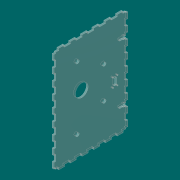
# Autodesk Inventor part: leftSide
Saved by Autodesk Inventor 2016 (Build 200138000, 138)
## iProperties
Created: 2015-10-05
Part Number: leftSide
Material: Polycarbonate, Clear
Document SubType Name: Modeling
Designer: Sawaiz
Density: 1.2 g/cm^3
Appearance: Polycarbonate - Clear
Author: Sawaiz
Autodesk Inventor part; units mm, degrees
ref_plane "YZ Plane" through (0, 0, 0) normal (1, 0, 0) x (0, 1, 0)
ref_plane "XZ Plane" through (0, 0, 0) normal (0, 1, 0) x (-1, 0, 0)
ref_plane "XY Plane" through (0, 0, 0) normal (0, 0, 1) x (1, 0, 0)
sketch "Sketch1" plane through (0, 0, 0) normal (1, 0, 0) x (0, 1, 0)
  line L0 (-60, -86.825) -> (60, -86.825)
  line L1 (60, -86.825) -> (60, 86.825)
  line L2 (60, 86.825) -> (-60, 86.825)
  line L3 (-60, 86.825) -> (-60, -86.825)
  line L4 (-60, -86.825) -> (60, 86.825) construction
  line L5 (60, -86.825) -> (-60, 86.825) construction
  point P0 (0, 0)
  dimension "d0" = 120
  dimension "d1" = 173.65
  constraints: 12 end point, 2 midpoint, 2 parallel, 1 horizontal, 1 perpendicular
  measures "d0" distance of L2.end L1.end
  measures "d1" distance of L1.end L0.end
extrude "Extrusion1" add sketch "Sketch1" along normal blind 3.175
sketch "Sketch10" plane through (0, 0, 0) normal (-1, 0, 0) x (0, 0, 1)
  line L0 (-86.825, -60) -> (-86.825, 60) projected
  line L1 (86.825, -60) -> (-86.825, -60) projected
  line L2 (86.825, 60) -> (86.825, -60) projected
  line L3 (-86.825, 60) -> (86.825, 60) projected
  line L4 (86.825, 60) -> (86.825, -60) projected
  line L5 (86.825, -55) -> (90, -55)
  line L6 (90, -55) -> (90, -45)
  line L7 (90, -45) -> (86.825, -45)
  line L8 (86.825, -45) -> (86.825, -55)
  point P0 (0, 0)
  dimension "d84" = 10
  dimension "d85" = 5
  dimension "d86" = 3.175
  constraints: 8 end point, 2 parallel, 1 horizontal, 1 perpendicular, 1 point on line
  measures "d84" distance of L5.end L6.end
  measures "d85" distance between parallel lines of L1 L5
  measures "d86" distance of L6.end L7.end
extrude "Extrusion4" add sketch "Sketch10" against normal up to surface (3.175 mm away) contours L2 L7 L6 L5
pattern_linear "Rectangular Pattern3" count 6 spacing 20 along (0, 1, 0) of "Extrusion4"
mirror "Mirror3" about plane through (0, 0, 0) normal (0, 0, 1) of "Extrusion4", "Rectangular Pattern3"
sketch "Sketch11" plane through (0, 0, 0) normal (-1, 0, 0) x (0, 0, 1)
  line L0 (-86.825, -60) -> (-86.825, -55) projected
  line L1 (86.825, -60) -> (-86.825, -60) projected
  line L2 (86.825, -55) -> (86.825, -60) projected
  line L3 (86.825, -55) -> (90, -55) projected
  line L4 (90, -55) -> (90, -45) projected
  line L5 (90, -45) -> (86.825, -45) projected
  line L6 (86.825, -35) -> (86.825, -45) projected
  line L7 (86.825, -35) -> (90, -35) projected
  line L8 (90, -35) -> (90, -25) projected
  line L9 (90, -25) -> (86.825, -25) projected
  line L10 (86.825, -15) -> (86.825, -25) projected
  line L11 (86.825, -15) -> (90, -15) projected
  line L12 (90, -15) -> (90, -5) projected
  line L13 (90, -5) -> (86.825, -5) projected
  line L14 (86.825, 5) -> (86.825, -5) projected
  line L15 (86.825, 5) -> (90, 5) projected
  line L16 (90, 5) -> (90, 15) projected
  line L17 (90, 15) -> (86.825, 15) projected
  line L18 (86.825, 25) -> (86.825, 15) projected
  line L19 (86.825, 25) -> (90, 25) projected
  line L20 (90, 25) -> (90, 35) projected
  line L21 (90, 35) -> (86.825, 35) projected
  line L22 (86.825, 45) -> (86.825, 35) projected
  line L23 (86.825, 45) -> (90, 45) projected
  line L24 (90, 45) -> (90, 55) projected
  line L25 (90, 55) -> (86.825, 55) projected
  line L26 (86.825, 60) -> (86.825, 55) projected
  line L27 (-86.825, 60) -> (86.825, 60) projected
  line L28 (-86.825, 55) -> (-86.825, 60) projected
  line L29 (-90, 55) -> (-86.825, 55) projected
  line L30 (-90, 45) -> (-90, 55) projected
  line L31 (-86.825, 45) -> (-90, 45) projected
  line L32 (-86.825, 35) -> (-86.825, 45) projected
  line L33 (-90, 35) -> (-86.825, 35) projected
  line L34 (-90, 25) -> (-90, 35) projected
  line L35 (-86.825, 25) -> (-90, 25) projected
  line L36 (-86.825, 15) -> (-86.825, 25) projected
  line L37 (-90, 15) -> (-86.825, 15) projected
  line L38 (-90, 5) -> (-90, 15) projected
  line L39 (-86.825, 5) -> (-90, 5) projected
  line L40 (-86.825, -5) -> (-86.825, 5) projected
  line L41 (-90, -5) -> (-86.825, -5) projected
  line L42 (-90, -15) -> (-90, -5) projected
  line L43 (-86.825, -15) -> (-90, -15) projected
  line L44 (-86.825, -25) -> (-86.825, -15) projected
  line L45 (-90, -25) -> (-86.825, -25) projected
  line L46 (-90, -35) -> (-90, -25) projected
  line L47 (-86.825, -35) -> (-90, -35) projected
  line L48 (-86.825, -45) -> (-86.825, -35) projected
  line L49 (-90, -45) -> (-86.825, -45) projected
  line L50 (-90, -55) -> (-90, -45) projected
  line L51 (-86.825, -55) -> (-90, -55) projected
  line L52 (86.825, -60) -> (-86.825, -60) projected
  line L53 (85, -60) -> (75, -60)
  line L54 (75, -60) -> (75, -63.175)
  line L55 (75, -63.175) -> (85, -63.175)
  line L56 (85, -63.175) -> (85, -60)
  point P0 (0, 0)
  dimension "d92" = 3.175
  dimension "d94" = 10
  dimension "d100" = 5
  constraints: 8 end point, 2 parallel, 1 horizontal, 1 perpendicular, 1 point on line
  measures "d92" distance of L55.end L53.start
  measures "d94" distance of L54.end L55.end
  measures "d100" distance between parallel lines of L4 L56
extrude "Extrusion5" add sketch "Sketch11" against normal up to surface (3.175 mm away) contours L1 L56 L55 L54
pattern_linear "Rectangular Pattern4" count 9 spacing 20 along (0, 0, -1) of "Extrusion5"
mirror "Mirror4" about plane through (0, 0, 0) normal (0, 1, 0) of "Extrusion5", "Rectangular Pattern4"
sketch "Sketch2" plane through (3.175, 0, 0) normal (1, 0, 0) x (0, 0, -1)
  line L0 (86.825, -60) -> (86.825, -55) projected
  line L1 (86.825, 60) -> (85, 60) projected
  line L2 (-86.825, 60) -> (-86.825, 55) projected
  line L3 (-86.825, -60) -> (-85, -60) projected
  line L4 (-86.825, 60) -> (-86.825, -60) projected
  line L5 (86.825, -55) -> (90, -55) projected
  line L6 (90, -55) -> (90, -45) projected
  line L7 (90, -45) -> (86.825, -45) projected
  line L8 (86.825, -45) -> (86.825, -35) projected
  line L9 (86.825, -35) -> (90, -35) projected
  line L10 (90, -35) -> (90, -25) projected
  line L11 (90, -25) -> (86.825, -25) projected
  line L12 (86.825, -25) -> (86.825, -15) projected
  line L13 (86.825, -15) -> (90, -15) projected
  line L14 (90, -15) -> (90, -5) projected
  line L15 (90, -5) -> (86.825, -5) projected
  line L16 (86.825, -5) -> (86.825, 5) projected
  line L17 (86.825, 5) -> (90, 5) projected
  line L18 (90, 5) -> (90, 15) projected
  line L19 (90, 15) -> (86.825, 15) projected
  line L20 (86.825, 15) -> (86.825, 25) projected
  line L21 (86.825, 25) -> (90, 25) projected
  line L22 (90, 25) -> (90, 35) projected
  line L23 (90, 35) -> (86.825, 35) projected
  line L24 (86.825, 35) -> (86.825, 45) projected
  line L25 (86.825, 45) -> (90, 45) projected
  line L26 (90, 45) -> (90, 55) projected
  line L27 (90, 55) -> (86.825, 55) projected
  line L28 (86.825, 55) -> (86.825, 60) projected
  line L29 (85, 60) -> (85, 63.175) projected
  line L30 (85, 63.175) -> (75, 63.175) projected
  line L31 (75, 63.175) -> (75, 60) projected
  line L32 (65, 60) -> (65, 63.175) projected
  line L33 (65, 63.175) -> (55, 63.175) projected
  line L34 (55, 63.175) -> (55, 60) projected
  line L35 (55, 60) -> (45, 60) projected
  line L36 (45, 60) -> (45, 63.175) projected
  line L37 (45, 63.175) -> (35, 63.175) projected
  line L38 (35, 63.175) -> (35, 60) projected
  line L39 (35, 60) -> (25, 60) projected
  line L40 (25, 60) -> (25, 63.175) projected
  line L41 (25, 63.175) -> (15, 63.175) projected
  line L42 (15, 63.175) -> (15, 60) projected
  line L43 (15, 60) -> (5, 60) projected
  line L44 (5, 60) -> (5, 63.175) projected
  line L45 (5, 63.175) -> (-5, 63.175) projected
  line L46 (-5, 63.175) -> (-5, 60) projected
  line L47 (-5, 60) -> (-15, 60) projected
  line L48 (-15, 60) -> (-15, 63.175) projected
  line L49 (-15, 63.175) -> (-25, 63.175) projected
  line L50 (-25, 63.175) -> (-25, 60) projected
  line L51 (-25, 60) -> (-35, 60) projected
  line L52 (-35, 60) -> (-35, 63.175) projected
  line L53 (-35, 63.175) -> (-45, 63.175) projected
  line L54 (-45, 63.175) -> (-45, 60) projected
  line L55 (-45, 60) -> (-55, 60) projected
  line L56 (-55, 60) -> (-55, 63.175) projected
  line L57 (-55, 63.175) -> (-65, 63.175) projected
  line L58 (-65, 63.175) -> (-65, 60) projected
  line L59 (-65, 60) -> (-75, 60) projected
  line L60 (-75, 60) -> (-75, 63.175) projected
  line L61 (-75, 63.175) -> (-85, 63.175) projected
  line L62 (-85, 63.175) -> (-85, 60) projected
  line L63 (-85, 60) -> (-86.825, 60) projected
  line L64 (-90, 55) -> (-86.825, 55) projected
  line L65 (-90, 45) -> (-90, 55) projected
  line L66 (-86.825, 45) -> (-90, 45) projected
  line L67 (-86.825, 45) -> (-86.825, 35) projected
  line L68 (-90, 35) -> (-86.825, 35) projected
  line L69 (-90, 25) -> (-90, 35) projected
  line L70 (-86.825, 25) -> (-90, 25) projected
  line L71 (-86.825, 25) -> (-86.825, 15) projected
  line L72 (-90, 15) -> (-86.825, 15) projected
  line L73 (-90, 5) -> (-90, 15) projected
  line L74 (-86.825, 5) -> (-90, 5) projected
  line L75 (-86.825, 5) -> (-86.825, -5) projected
  line L76 (-90, -5) -> (-86.825, -5) projected
  line L77 (-90, -15) -> (-90, -5) projected
  line L78 (-86.825, -15) -> (-90, -15) projected
  line L79 (-86.825, -15) -> (-86.825, -25) projected
  line L80 (-90, -25) -> (-86.825, -25) projected
  line L81 (-90, -35) -> (-90, -25) projected
  line L82 (-86.825, -35) -> (-90, -35) projected
  line L83 (-86.825, -35) -> (-86.825, -45) projected
  line L84 (-90, -45) -> (-86.825, -45) projected
  line L85 (-90, -55) -> (-90, -45) projected
  line L86 (-86.825, -55) -> (-90, -55) projected
  line L87 (-86.825, -55) -> (-86.825, -60) projected
  line L88 (-85, -63.175) -> (-85, -60) projected
  line L89 (-75, -63.175) -> (-85, -63.175) projected
  line L90 (-75, -60) -> (-75, -63.175) projected
  line L91 (-75, -60) -> (-65, -60) projected
  line L92 (-65, -63.175) -> (-65, -60) projected
  line L93 (-55, -63.175) -> (-65, -63.175) projected
  line L94 (-55, -60) -> (-55, -63.175) projected
  line L95 (-55, -60) -> (-45, -60) projected
  line L96 (-45, -63.175) -> (-45, -60) projected
  line L97 (-35, -63.175) -> (-45, -63.175) projected
  line L98 (-35, -60) -> (-35, -63.175) projected
  line L99 (-35, -60) -> (-25, -60) projected
  line L100 (-25, -63.175) -> (-25, -60) projected
  line L101 (-15, -63.175) -> (-25, -63.175) projected
  line L102 (-15, -60) -> (-15, -63.175) projected
  line L103 (-15, -60) -> (-5, -60) projected
  line L104 (-5, -63.175) -> (-5, -60) projected
  line L105 (5, -63.175) -> (-5, -63.175) projected
  line L106 (5, -60) -> (5, -63.175) projected
  line L107 (5, -60) -> (15, -60) projected
  line L108 (15, -63.175) -> (15, -60) projected
  line L109 (25, -63.175) -> (15, -63.175) projected
  line L110 (25, -60) -> (25, -63.175) projected
  line L111 (25, -60) -> (35, -60) projected
  line L112 (35, -63.175) -> (35, -60) projected
  line L113 (45, -63.175) -> (35, -63.175) projected
  line L114 (45, -60) -> (45, -63.175) projected
  line L115 (45, -60) -> (55, -60) projected
  line L116 (55, -63.175) -> (55, -60) projected
  line L117 (65, -63.175) -> (55, -63.175) projected
  line L118 (65, -60) -> (65, -63.175) projected
  line L119 (65, -60) -> (75, -60) projected
  line L120 (75, -63.175) -> (75, -60) projected
  line L121 (85, -63.175) -> (75, -63.175) projected
  line L122 (85, -60) -> (85, -63.175) projected
  line L123 (75, 60) -> (65, 60) projected
  line L124 (85, -60) -> (86.825, -60) projected
  point P0 (0, 0)
  point P1 (-8.175, -15.675)
  dimension "d4" = 95
  dimension "d12" = 44.325
  measures "d4" distance from line of L0 point (-8.175, -15.675)
  measures "d12" distance from line of L3 point (-8.175, -15.675)
hole "Hole1" at (3.175, -15.675, 8.175) direction (-1, 0, 0) diameter 22 end through all
sketch "Sketch6" plane through (3.175, 0, 0) normal (1, 0, 0) x (0, 0, -1)
  circle A0 centre (-8.175, -15.675) radius 11 projected
  line L0 (86.825, -60) -> (86.825, -55) projected
  line L1 (86.825, 60) -> (85, 60) projected
  line L2 (-86.825, 60) -> (-86.825, 55) projected
  line L3 (-86.825, -60) -> (-85, -60) projected
  line L4 (-86.825, -60) -> (86.825, -60) projected
  line L5 (-48.5, 60) -> (-48.5, 58)
  line L6 (-48.5, 58) -> (-47.25, 58)
  line L7 (-47.25, 58) -> (-47.25, 55.5)
  line L8 (-47.25, 55.5) -> (-48.5, 55.5)
  line L9 (-48.5, 55.5) -> (-48.5, 49.175)
  line L10 (-48.5, 49.175) -> (-51.5, 49.175)
  line L11 (-51.5, 49.175) -> (-51.5, 55.5)
  line L12 (-51.5, 55.5) -> (-52.75, 55.5)
  line L13 (-52.75, 55.5) -> (-52.75, 58)
  line L14 (-52.75, 58) -> (-51.5, 58)
  line L15 (-51.5, 60) -> (-51.5, 58)
  line L16 (86.825, -55) -> (90, -55) projected
  line L17 (90, -55) -> (90, -45) projected
  line L18 (90, -45) -> (86.825, -45) projected
  line L19 (86.825, -45) -> (86.825, -35) projected
  line L20 (86.825, -35) -> (90, -35) projected
  line L21 (90, -35) -> (90, -25) projected
  line L22 (90, -25) -> (86.825, -25) projected
  line L23 (86.825, -25) -> (86.825, -15) projected
  line L24 (86.825, -15) -> (90, -15) projected
  line L25 (90, -15) -> (90, -5) projected
  line L26 (90, -5) -> (86.825, -5) projected
  line L27 (86.825, -5) -> (86.825, 5) projected
  line L28 (86.825, 5) -> (90, 5) projected
  line L29 (90, 5) -> (90, 15) projected
  line L30 (90, 15) -> (86.825, 15) projected
  line L31 (86.825, 15) -> (86.825, 25) projected
  line L32 (86.825, 25) -> (90, 25) projected
  line L33 (90, 25) -> (90, 35) projected
  line L34 (90, 35) -> (86.825, 35) projected
  line L35 (86.825, 35) -> (86.825, 45) projected
  line L36 (86.825, 45) -> (90, 45) projected
  line L37 (90, 45) -> (90, 55) projected
  line L38 (90, 55) -> (86.825, 55) projected
  line L39 (85, 60) -> (85, 63.175) projected
  line L40 (85, 63.175) -> (75, 63.175) projected
  line L41 (75, 63.175) -> (75, 60) projected
  line L42 (75, 60) -> (65, 60) projected
  line L43 (65, 60) -> (65, 63.175) projected
  line L44 (65, 63.175) -> (55, 63.175) projected
  line L45 (55, 63.175) -> (55, 60) projected
  line L46 (55, 60) -> (45, 60) projected
  line L47 (45, 60) -> (45, 63.175) projected
  line L48 (45, 63.175) -> (35, 63.175) projected
  line L49 (35, 63.175) -> (35, 60) projected
  line L50 (25, 60) -> (25, 63.175) projected
  line L51 (25, 63.175) -> (15, 63.175) projected
  line L52 (15, 63.175) -> (15, 60) projected
  line L53 (15, 60) -> (5, 60) projected
  line L54 (5, 60) -> (5, 63.175) projected
  line L55 (5, 63.175) -> (-5, 63.175) projected
  line L56 (-5, 63.175) -> (-5, 60) projected
  line L57 (-5, 60) -> (-15, 60) projected
  line L58 (-15, 60) -> (-15, 63.175) projected
  line L59 (-15, 63.175) -> (-25, 63.175) projected
  line L60 (-25, 63.175) -> (-25, 60) projected
  line L61 (-25, 60) -> (-35, 60) projected
  line L62 (-35, 60) -> (-35, 63.175) projected
  line L63 (-35, 63.175) -> (-45, 63.175) projected
  line L64 (-45, 63.175) -> (-45, 60) projected
  line L65 (-45, 60) -> (-55, 60) projected
  line L66 (-55, 60) -> (-55, 63.175) projected
  line L67 (-55, 63.175) -> (-65, 63.175) projected
  line L68 (-65, 63.175) -> (-65, 60) projected
  line L69 (-65, 60) -> (-75, 60) projected
  line L70 (-75, 60) -> (-75, 63.175) projected
  line L71 (-75, 63.175) -> (-85, 63.175) projected
  line L72 (-85, 63.175) -> (-85, 60) projected
  line L73 (-85, 60) -> (-86.825, 60) projected
  line L74 (-90, 55) -> (-86.825, 55) projected
  line L75 (-90, 45) -> (-90, 55) projected
  line L76 (-86.825, 45) -> (-90, 45) projected
  line L77 (-86.825, 45) -> (-86.825, 35) projected
  line L78 (-90, 35) -> (-86.825, 35) projected
  line L79 (-90, 25) -> (-90, 35) projected
  line L80 (-86.825, 25) -> (-90, 25) projected
  line L81 (-90, 15) -> (-86.825, 15) projected
  line L82 (-90, 5) -> (-90, 15) projected
  line L83 (-86.825, 5) -> (-90, 5) projected
  line L84 (-86.825, 5) -> (-86.825, -5) projected
  line L85 (-90, -5) -> (-86.825, -5) projected
  line L86 (-90, -15) -> (-90, -5) projected
  line L87 (-86.825, -15) -> (-90, -15) projected
  line L88 (-86.825, -15) -> (-86.825, -25) projected
  line L89 (-90, -25) -> (-86.825, -25) projected
  line L90 (-90, -35) -> (-90, -25) projected
  line L91 (-86.825, -35) -> (-90, -35) projected
  line L92 (-86.825, -35) -> (-86.825, -45) projected
  line L93 (-90, -45) -> (-86.825, -45) projected
  line L94 (-90, -55) -> (-90, -45) projected
  line L95 (-86.825, -55) -> (-90, -55) projected
  line L96 (-86.825, -55) -> (-86.825, -60) projected
  line L97 (-85, -63.175) -> (-85, -60) projected
  line L98 (-75, -63.175) -> (-85, -63.175) projected
  line L99 (-75, -60) -> (-75, -63.175) projected
  line L100 (-75, -60) -> (-65, -60) projected
  line L101 (-65, -63.175) -> (-65, -60) projected
  line L102 (-55, -63.175) -> (-65, -63.175) projected
  line L103 (-55, -60) -> (-55, -63.175) projected
  line L104 (-55, -60) -> (-45, -60) projected
  line L105 (-45, -63.175) -> (-45, -60) projected
  line L106 (-35, -63.175) -> (-45, -63.175) projected
  line L107 (-35, -60) -> (-35, -63.175) projected
  line L108 (-35, -60) -> (-25, -60) projected
  line L109 (-25, -63.175) -> (-25, -60) projected
  line L110 (-15, -63.175) -> (-25, -63.175) projected
  line L111 (-15, -60) -> (-15, -63.175) projected
  line L112 (-5, -63.175) -> (-5, -60) projected
  line L113 (5, -63.175) -> (-5, -63.175) projected
  line L114 (5, -60) -> (5, -63.175) projected
  line L115 (5, -60) -> (15, -60) projected
  line L116 (15, -63.175) -> (15, -60) projected
  line L117 (25, -63.175) -> (15, -63.175) projected
  line L118 (25, -60) -> (25, -63.175) projected
  line L119 (25, -60) -> (35, -60) projected
  line L120 (35, -63.175) -> (35, -60) projected
  line L121 (45, -63.175) -> (35, -63.175) projected
  line L122 (45, -60) -> (45, -63.175) projected
  line L123 (45, -60) -> (55, -60) projected
  line L124 (55, -63.175) -> (55, -60) projected
  line L125 (65, -63.175) -> (55, -63.175) projected
  line L126 (65, -60) -> (65, -63.175) projected
  line L127 (65, -60) -> (75, -60) projected
  line L128 (75, -63.175) -> (75, -60) projected
  line L129 (85, -63.175) -> (75, -63.175) projected
  line L130 (85, -60) -> (85, -63.175) projected
  line L131 (-86.825, 25) -> (-86.825, 15) projected
  line L132 (-15, -60) -> (-5, -60) projected
  line L133 (-51.5, 60) -> (-48.5, 60)
  line L134 (86.825, 55) -> (86.825, 60) projected
  line L135 (35, 60) -> (25, 60) projected
  line L136 (85, -60) -> (86.825, -60) projected
  point P0 (0, 0)
  point P1 (-50, 49.175)
  dimension "d40" = 3
  dimension "d41" = 5.5
  dimension "d42" = 2.5
  dimension "d101" = 10.825
  dimension "d103" = 2
  dimension "d104" = 2
  dimension "d105" = 50
  constraints: 24 end point, 8 point on line, 6 perpendicular, 1 collinear, 1 midpoint, 1 vertical
  measures "d40" distance between parallel lines of L15 L5
  measures "d41" distance between parallel lines of L7 L13
  measures "d42" distance between parallel lines of L14 L12
  measures "d101" distance from line of L5.start L10
  measures "d103" distance from line of L14 L15.start
  measures "d104" distance from line of L5.start L6
  measures "d105" horizontal distance of point (0, 0) point (-50, 49.175)
sketch "Sketch9" plane through (3.175, 0, 0) normal (1, 0, 0) x (0, 0, -1)
  line L0 (54, -22.9972) -> (-54, -22.9972)
  line L1 (-54, -22.9972) -> (-27.4451, 22.9972)
  line L2 (-27.4451, 22.9972) -> (27.4451, 22.9972)
  line L3 (27.4451, 22.9972) -> (54, -22.9972)
  line L4 (-45, -63.175) -> (-45, -60) projected
  line L5 (-35, -63.175) -> (-45, -63.175) projected
  line L6 (-35, -60) -> (-35, -63.175) projected
  line L7 (-25, -63.175) -> (-25, -60) projected
  line L8 (-15, -63.175) -> (-25, -63.175) projected
  line L9 (-15, -60) -> (-15, -63.175) projected
  line L10 (-5, -63.175) -> (-5, -60) projected
  line L11 (5, -63.175) -> (-5, -63.175) projected
  line L12 (5, -60) -> (5, -63.175) projected
  line L13 (15, -63.175) -> (15, -60) projected
  line L14 (25, -63.175) -> (15, -63.175) projected
  line L15 (25, -60) -> (25, -63.175) projected
  line L16 (35, -63.175) -> (35, -60) projected
  line L17 (45, -63.175) -> (35, -63.175) projected
  line L18 (45, -60) -> (45, -63.175) projected
  line L19 (55, -63.175) -> (55, -60) projected
  line L20 (65, -63.175) -> (55, -63.175) projected
  line L21 (65, -60) -> (65, -63.175) projected
  line L22 (75, -63.175) -> (75, -60) projected
  line L23 (85, -63.175) -> (75, -63.175) projected
  line L24 (85, -60) -> (85, -63.175) projected
  line L25 (-85, -63.175) -> (-85, -60) projected
  line L26 (-75, -63.175) -> (-85, -63.175) projected
  line L27 (-75, -60) -> (-75, -63.175) projected
  line L28 (-65, -63.175) -> (-65, -60) projected
  line L29 (-55, -63.175) -> (-65, -63.175) projected
  line L30 (-55, -60) -> (-55, -63.175) projected
  line L31 (86.825, -60) -> (86.825, -55) projected
  line L32 (86.825, -55) -> (90, -55) projected
  line L33 (90, -55) -> (90, -45) projected
  line L34 (90, -45) -> (86.825, -45) projected
  line L35 (86.825, -45) -> (86.825, -35) projected
  line L36 (86.825, -35) -> (90, -35) projected
  line L37 (90, -35) -> (90, -25) projected
  line L38 (90, -25) -> (86.825, -25) projected
  line L39 (86.825, -25) -> (86.825, -15) projected
  line L40 (86.825, -15) -> (90, -15) projected
  line L41 (90, -15) -> (90, -5) projected
  line L42 (90, -5) -> (86.825, -5) projected
  line L43 (86.825, -5) -> (86.825, 5) projected
  line L44 (86.825, 5) -> (90, 5) projected
  line L45 (90, 5) -> (90, 15) projected
  line L46 (90, 15) -> (86.825, 15) projected
  line L47 (86.825, 15) -> (86.825, 25) projected
  line L48 (86.825, 25) -> (90, 25) projected
  line L49 (90, 25) -> (90, 35) projected
  line L50 (90, 35) -> (86.825, 35) projected
  line L51 (86.825, 35) -> (86.825, 45) projected
  line L52 (86.825, 45) -> (90, 45) projected
  line L53 (90, 45) -> (90, 55) projected
  line L54 (90, 55) -> (86.825, 55) projected
  line L55 (86.825, 55) -> (86.825, 60) projected
  line L56 (86.825, 60) -> (85, 60) projected
  line L57 (85, 60) -> (85, 63.175) projected
  line L58 (85, 63.175) -> (75, 63.175) projected
  line L59 (75, 63.175) -> (75, 60) projected
  line L60 (75, 60) -> (65, 60) projected
  line L61 (65, 60) -> (65, 63.175) projected
  line L62 (65, 63.175) -> (55, 63.175) projected
  line L63 (55, 63.175) -> (55, 60) projected
  line L64 (55, 60) -> (45, 60) projected
  line L65 (45, 60) -> (45, 63.175) projected
  line L66 (45, 63.175) -> (35, 63.175) projected
  line L67 (35, 63.175) -> (35, 60) projected
  line L68 (35, 60) -> (25, 60) projected
  line L69 (25, 60) -> (25, 63.175) projected
  line L70 (25, 63.175) -> (15, 63.175) projected
  line L71 (15, 63.175) -> (15, 60) projected
  line L72 (15, 60) -> (5, 60) projected
  line L73 (5, 60) -> (5, 63.175) projected
  line L74 (5, 63.175) -> (-5, 63.175) projected
  line L75 (-5, 63.175) -> (-5, 60) projected
  line L76 (-5, 60) -> (-15, 60) projected
  line L77 (-15, 60) -> (-15, 63.175) projected
  line L78 (-15, 63.175) -> (-25, 63.175) projected
  line L79 (-25, 63.175) -> (-25, 60) projected
  line L80 (-25, 60) -> (-35, 60) projected
  line L81 (-35, 60) -> (-35, 63.175) projected
  line L82 (-35, 63.175) -> (-45, 63.175) projected
  line L83 (-45, 63.175) -> (-45, 60) projected
  line L84 (-45, 60) -> (-55, 60) projected
  line L85 (-55, 60) -> (-55, 63.175) projected
  line L86 (-55, 63.175) -> (-65, 63.175) projected
  line L87 (-65, 63.175) -> (-65, 60) projected
  line L88 (-65, 60) -> (-75, 60) projected
  line L89 (-75, 60) -> (-75, 63.175) projected
  line L90 (-75, 63.175) -> (-85, 63.175) projected
  line L91 (-85, 63.175) -> (-85, 60) projected
  line L92 (-85, 60) -> (-86.825, 60) projected
  line L93 (-86.825, 60) -> (-86.825, 55) projected
  line L94 (-90, 55) -> (-86.825, 55) projected
  line L95 (-90, 45) -> (-90, 55) projected
  line L96 (-86.825, 45) -> (-90, 45) projected
  line L97 (-86.825, 45) -> (-86.825, 35) projected
  line L98 (-90, 35) -> (-86.825, 35) projected
  line L99 (-90, 25) -> (-90, 35) projected
  line L100 (-86.825, 25) -> (-90, 25) projected
  line L101 (-86.825, 25) -> (-86.825, 15) projected
  line L102 (-90, 15) -> (-86.825, 15) projected
  line L103 (-90, 5) -> (-90, 15) projected
  line L104 (-86.825, 5) -> (-90, 5) projected
  line L105 (-86.825, 5) -> (-86.825, -5) projected
  line L106 (-90, -5) -> (-86.825, -5) projected
  line L107 (-90, -15) -> (-90, -5) projected
  line L108 (-86.825, -15) -> (-90, -15) projected
  line L109 (-86.825, -15) -> (-86.825, -25) projected
  line L110 (-90, -25) -> (-86.825, -25) projected
  line L111 (-90, -35) -> (-90, -25) projected
  line L112 (-86.825, -35) -> (-90, -35) projected
  line L113 (-86.825, -35) -> (-86.825, -45) projected
  line L114 (-90, -45) -> (-86.825, -45) projected
  line L115 (-90, -55) -> (-90, -45) projected
  line L116 (-86.825, -55) -> (-90, -55) projected
  line L117 (-86.825, -55) -> (-86.825, -60) projected
  line L118 (-86.825, -60) -> (-85, -60) projected
  line L119 (-75, -60) -> (-65, -60) projected
  line L120 (-55, -60) -> (-45, -60) projected
  line L121 (-35, -60) -> (-25, -60) projected
  line L122 (-15, -60) -> (-5, -60) projected
  line L123 (5, -60) -> (15, -60) projected
  line L124 (25, -60) -> (35, -60) projected
  line L125 (45, -60) -> (55, -60) projected
  line L126 (65, -60) -> (75, -60) projected
  line L127 (85, -60) -> (86.825, -60) projected
  point P0 (0, 0)
  dimension "d74" = 60
  dimension "d75" = 60
  constraints: 8 end point, 2 horizontal
  measures "d74" angle of L0 L1
  measures "d75" angle of L0 L3
hole "Hole6" at (3.175, -22.9972, 54) at (3.175, 22.9972, 27.4451) at (3.175, 22.9972, -27.4451) at (3.175, -22.9972, -54) direction (-1, 0, 0) diameter 6 end through all
extrude "Extrusion6" cut sketch "Sketch6" against normal through all contours L65 L5 L6 L7 L8 L9 L10 L11 L12 L13 L14 L15
mirror "Mirror5" about plane through (0, 0, 0) normal (0, 0, 1) of "Extrusion6"
sketch "Sketch14" plane through (0, 0, 0) normal (-1, 0, 0) x (0, 0, 1)
  line L0 (-15.24, 45.72) -> (0, 45.72) construction
  line L1 (0, 45.72) -> (0, 0) construction
  line L2 (-15.24, 38.1) -> (-15.24, 45.72) construction
  line L3 (-15.24, 38.1) -> (0, 38.1) construction
  dimension "d127" = 45.72
  dimension "d128" = 15.24
  dimension "d142" = 7.62
  constraints: 8 end point, 2 horizontal, 1 perpendicular, 1 point on line, 1 vertical
  measures "d127" distance of L0.end L1.end
  measures "d128" distance of L0.start L0.end
  measures "d142" distance of L2.start L0.start
hole "Hole9" at (0, 45.72, 0) at (0, 45.72, -15.24) at (0, 38.1, -15.24) at (0, 38.1, 0) direction (1, 0, 0) diameter 2.156 end through all thread size "4-40 UNC" class "2B" standard "ANSI Unified Screw Threads"
sketch "Sketch15" plane through (0, 0, 0) normal (-1, 0, 0) x (0, 0, 1)
  line L0 (-1.905, 43.815) -> (-13.335, 43.815)
  line L1 (-13.335, 43.815) -> (-13.335, 40.005)
  line L2 (-13.335, 40.005) -> (-1.905, 40.005)
  line L3 (-1.905, 40.005) -> (-1.905, 43.815)
  circle A0 centre (0, 45.72) radius 1.078 projected
  circle A1 centre (-15.24, 45.72) radius 1.078 projected
  circle A2 centre (-27.4451, 22.9972) radius 3 projected
  circle A3 centre (54, -22.9972) radius 3 projected
  circle A4 centre (27.4451, 22.9972) radius 3 projected
  circle A5 centre (-54, -22.9972) radius 3 projected
  circle A6 centre (8.175, -15.675) radius 11 projected
  line L4 (-48.5, 60) -> (-48.5, 58) projected
  line L5 (-48.5, 58) -> (-47.25, 58) projected
  line L6 (-47.25, 58) -> (-47.25, 55.5) projected
  line L7 (-47.25, 55.5) -> (-48.5, 55.5) projected
  line L8 (-48.5, 55.5) -> (-48.5, 49.175) projected
  line L9 (-48.5, 49.175) -> (-51.5, 49.175) projected
  line L10 (-51.5, 49.175) -> (-51.5, 55.5) projected
  line L11 (-51.5, 55.5) -> (-52.75, 55.5) projected
  line L12 (-52.75, 55.5) -> (-52.75, 58) projected
  line L13 (-52.75, 58) -> (-51.5, 58) projected
  line L14 (-51.5, 58) -> (-51.5, 60) projected
  line L15 (-55, 60) -> (-51.5, 60) projected
  line L16 (-55, 63.175) -> (-55, 60) projected
  line L17 (-65, 63.175) -> (-55, 63.175) projected
  line L18 (-65, 60) -> (-65, 63.175) projected
  line L19 (-75, 60) -> (-65, 60) projected
  line L20 (-75, 63.175) -> (-75, 60) projected
  line L21 (-85, 63.175) -> (-75, 63.175) projected
  line L22 (-85, 60) -> (-85, 63.175) projected
  line L23 (-86.825, 60) -> (-85, 60) projected
  line L24 (-86.825, 55) -> (-86.825, 60) projected
  line L25 (-90, 55) -> (-86.825, 55) projected
  line L26 (-90, 45) -> (-90, 55) projected
  line L27 (-86.825, 45) -> (-90, 45) projected
  line L28 (-86.825, 35) -> (-86.825, 45) projected
  line L29 (-90, 35) -> (-86.825, 35) projected
  line L30 (-90, 25) -> (-90, 35) projected
  line L31 (-86.825, 25) -> (-90, 25) projected
  line L32 (-86.825, 15) -> (-86.825, 25) projected
  line L33 (-90, 15) -> (-86.825, 15) projected
  line L34 (-90, 5) -> (-90, 15) projected
  line L35 (-86.825, 5) -> (-90, 5) projected
  line L36 (-86.825, -5) -> (-86.825, 5) projected
  line L37 (-90, -5) -> (-86.825, -5) projected
  line L38 (-90, -15) -> (-90, -5) projected
  line L39 (-86.825, -15) -> (-90, -15) projected
  line L40 (-86.825, -25) -> (-86.825, -15) projected
  line L41 (-90, -25) -> (-86.825, -25) projected
  line L42 (-90, -35) -> (-90, -25) projected
  line L43 (-86.825, -35) -> (-90, -35) projected
  line L44 (-86.825, -45) -> (-86.825, -35) projected
  line L45 (-90, -45) -> (-86.825, -45) projected
  line L46 (-90, -55) -> (-90, -45) projected
  line L47 (-86.825, -55) -> (-90, -55) projected
  line L48 (-86.825, -60) -> (-86.825, -55) projected
  line L49 (-85, -60) -> (-86.825, -60) projected
  line L50 (-85, -60) -> (-85, -63.175) projected
  line L51 (-85, -63.175) -> (-75, -63.175) projected
  line L52 (-75, -63.175) -> (-75, -60) projected
  line L53 (-65, -60) -> (-75, -60) projected
  line L54 (-65, -60) -> (-65, -63.175) projected
  line L55 (-65, -63.175) -> (-55, -63.175) projected
  line L56 (-55, -63.175) -> (-55, -60) projected
  line L57 (-45, -60) -> (-55, -60) projected
  line L58 (-45, -60) -> (-45, -63.175) projected
  line L59 (-45, -63.175) -> (-35, -63.175) projected
  line L60 (-35, -63.175) -> (-35, -60) projected
  line L61 (-25, -60) -> (-35, -60) projected
  line L62 (-25, -60) -> (-25, -63.175) projected
  line L63 (-25, -63.175) -> (-15, -63.175) projected
  line L64 (-15, -63.175) -> (-15, -60) projected
  line L65 (-5, -60) -> (-15, -60) projected
  line L66 (-5, -60) -> (-5, -63.175) projected
  line L67 (-5, -63.175) -> (5, -63.175) projected
  line L68 (5, -63.175) -> (5, -60) projected
  line L69 (15, -60) -> (5, -60) projected
  line L70 (15, -60) -> (15, -63.175) projected
  line L71 (15, -63.175) -> (25, -63.175) projected
  line L72 (25, -63.175) -> (25, -60) projected
  line L73 (35, -60) -> (25, -60) projected
  line L74 (35, -60) -> (35, -63.175) projected
  line L75 (35, -63.175) -> (45, -63.175) projected
  line L76 (45, -63.175) -> (45, -60) projected
  line L77 (55, -60) -> (45, -60) projected
  line L78 (55, -60) -> (55, -63.175) projected
  line L79 (55, -63.175) -> (65, -63.175) projected
  line L80 (65, -63.175) -> (65, -60) projected
  line L81 (75, -60) -> (65, -60) projected
  line L82 (75, -60) -> (75, -63.175) projected
  line L83 (75, -63.175) -> (85, -63.175) projected
  line L84 (85, -63.175) -> (85, -60) projected
  line L85 (86.825, -60) -> (85, -60) projected
  line L86 (86.825, -55) -> (86.825, -60) projected
  line L87 (86.825, -55) -> (90, -55) projected
  line L88 (90, -55) -> (90, -45) projected
  line L89 (90, -45) -> (86.825, -45) projected
  line L90 (86.825, -35) -> (86.825, -45) projected
  line L91 (86.825, -35) -> (90, -35) projected
  line L92 (90, -35) -> (90, -25) projected
  line L93 (90, -25) -> (86.825, -25) projected
  line L94 (86.825, -15) -> (86.825, -25) projected
  line L95 (86.825, -15) -> (90, -15) projected
  line L96 (90, -15) -> (90, -5) projected
  line L97 (90, -5) -> (86.825, -5) projected
  line L98 (86.825, 5) -> (86.825, -5) projected
  line L99 (86.825, 5) -> (90, 5) projected
  line L100 (90, 5) -> (90, 15) projected
  line L101 (90, 15) -> (86.825, 15) projected
  line L102 (86.825, 25) -> (86.825, 15) projected
  line L103 (86.825, 25) -> (90, 25) projected
  line L104 (90, 25) -> (90, 35) projected
  line L105 (90, 35) -> (86.825, 35) projected
  line L106 (86.825, 45) -> (86.825, 35) projected
  line L107 (86.825, 45) -> (90, 45) projected
  line L108 (90, 45) -> (90, 55) projected
  line L109 (90, 55) -> (86.825, 55) projected
  line L110 (86.825, 60) -> (86.825, 55) projected
  line L111 (85, 60) -> (86.825, 60) projected
  line L112 (85, 63.175) -> (85, 60) projected
  line L113 (75, 63.175) -> (85, 63.175) projected
  line L114 (75, 60) -> (75, 63.175) projected
  line L115 (65, 60) -> (75, 60) projected
  line L116 (65, 63.175) -> (65, 60) projected
  line L117 (55, 63.175) -> (65, 63.175) projected
  line L118 (55, 60) -> (55, 63.175) projected
  line L119 (51.5, 60) -> (55, 60) projected
  line L120 (51.5, 60) -> (51.5, 58) projected
  line L121 (51.5, 58) -> (52.75, 58) projected
  line L122 (52.75, 58) -> (52.75, 55.5) projected
  line L123 (52.75, 55.5) -> (51.5, 55.5) projected
  line L124 (51.5, 55.5) -> (51.5, 49.175) projected
  line L125 (51.5, 49.175) -> (48.5, 49.175) projected
  line L126 (48.5, 49.175) -> (48.5, 55.5) projected
  line L127 (48.5, 55.5) -> (47.25, 55.5) projected
  line L128 (47.25, 55.5) -> (47.25, 58) projected
  line L129 (47.25, 58) -> (48.5, 58) projected
  line L130 (48.5, 58) -> (48.5, 60) projected
  line L131 (45, 60) -> (48.5, 60) projected
  line L132 (45, 63.175) -> (45, 60) projected
  line L133 (35, 63.175) -> (45, 63.175) projected
  line L134 (35, 60) -> (35, 63.175) projected
  line L135 (25, 60) -> (35, 60) projected
  line L136 (25, 63.175) -> (25, 60) projected
  line L137 (15, 63.175) -> (25, 63.175) projected
  line L138 (15, 60) -> (15, 63.175) projected
  line L139 (5, 60) -> (15, 60) projected
  line L140 (5, 63.175) -> (5, 60) projected
  line L141 (-5, 63.175) -> (5, 63.175) projected
  line L142 (-5, 60) -> (-5, 63.175) projected
  line L143 (-15, 60) -> (-5, 60) projected
  line L144 (-15, 63.175) -> (-15, 60) projected
  line L145 (-25, 63.175) -> (-15, 63.175) projected
  line L146 (-25, 60) -> (-25, 63.175) projected
  line L147 (-35, 60) -> (-25, 60) projected
  line L148 (-35, 63.175) -> (-35, 60) projected
  line L149 (-45, 63.175) -> (-35, 63.175) projected
  line L150 (-45, 60) -> (-45, 63.175) projected
  line L151 (-48.5, 60) -> (-45, 60) projected
  point P0 (0, 0)
  dimension "d136" = 1.905
  dimension "d137" = 1.905
  dimension "d138" = 11.43
  dimension "d139" = 3.81
  constraints: 8 end point, 2 parallel, 1 horizontal, 1 perpendicular
  measures "d136" distance from line of A0.centre L3
  measures "d137" distance from line of A0.centre L0
  measures "d138" distance of L0.start L0.end
  measures "d139" distance of L0.end L1.end
extrude "Extrusion7" cut sketch "Sketch15" against normal through all contours L3 L2 L1 L0
equation "\"d0\" = depth"
equation "\"d1\" = height - 2 * materialThickness"
equation "\"d2\" = materialThickness"
equation "\"d84\" = notchWidth"
equation "\"d85\" = 0.5 * notchWidth"
equation "\"d86\" = materialThickness"
equation "\"d91\" = 2 * notchWidth"
equation "\"d92\" = materialThickness"
equation "\"d94\" = notchWidth"
equation "\"d100\" = 0.5 * notchWidth"
equation "\"d99\" = 2 * notchWidth"
equation "\"d4\" = axleHeight"
equation "\"d12\" = 0.5 * spoolDiameter - materialThickness"
equation "\"d5\" = bearingOd"
equation "\"d41\" = nutTrapwidth"
equation "\"d42\" = nutTrapDepth"
equation "\"d77\" = magnetDiameter"
equation "\"depth\" = 120"
equation "\"materialThickness\" = 3.175"
equation "\"laserKerf\" = 0.1"
equation "\"cardPinDiameter\" = 3"
equation "\"spoolDiameter\" = 95"
equation "\"cardHeight\" = 53.98"
equation "\"cardSelected\" = 1"
equation "\"cardFillet\" = 2.88"
equation "\"centeralShaftDiameter\" = 8"
equation "\"cardThickness\" = 0.76"
equation "\"cardWidth\" = 85.6"
equation "\"cardClearence\" = 0.5"
equation "\"bearingWidth\" = 8"
equation "\"bearingOd\" = 22"
equation "\"axleHeight\" = 95"
equation "\"nutTrapDepth\" = 2.5"
equation "\"nutTrapClearence\" = 2"
equation "\"nutTrapwidth\" = 5.5"
equation "\"magnetLength\" = 3"
equation "\"magnetDiameter\" = 6"
equation "\"magnetProtusion\" = 0.25"
equation "\"notchWidth\" = 10"
equation "\"spoolThickness\" = 5.588"
equation "\"height\" = 180"
body "Solid1"
